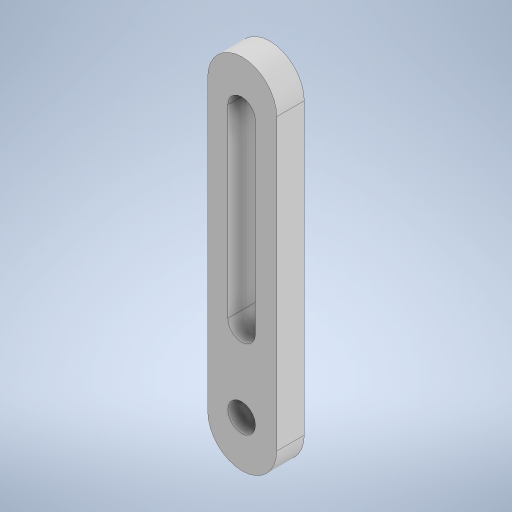
# Autodesk Inventor part: фанерная качалка
Saved by Autodesk Inventor 2023 (Build 270158000, 158)
## iProperties
Created: 2024-03-19
Part Number: фанерная качалка
Material: Типовые
Document SubType Name: Modeling
Designer: liza
Density: 1 g/cm^3
Appearance: По умолчанию
Author: liza
Autodesk Inventor part; units mm, degrees
ref_plane "YZ Plane" through (0, 0, 0) normal (1, 0, 0) x (0, 1, 0)
ref_plane "XZ Plane" through (0, 0, 0) normal (0, 1, 0) x (-1, 0, 0)
ref_plane "XY Plane" through (0, 0, 0) normal (0, 0, 1) x (1, 0, 0)
sketch "Эскиз1" plane through (0, 0, 0) normal (0, 0, 1) x (1, 0, 0)
  arc A0 (7.9627, -8) -> (-2.0373, -8) centre (2.9627, -8) ccw
  line L0 (-2.0373, -8) -> (-2.0373, -50)
  line L1 (7.9627, -8) -> (7.9627, -50)
  arc A1 (-2.0373, -50) -> (7.9627, -50) centre (2.9627, -50) ccw
  dimension "d7" = 42
  dimension "d8" = 5
  constraints: 4 end point, 4 point on circle, 4 tangent, 2 centre point, 2 vertical
  measures "d7" distance of L1.start L1.end
  measures "d8" radius of A1
extrude "Выдавливание1" add sketch "Эскиз1" along normal blind 4
sketch "Эскиз2" plane through (0, 0, 4) normal (0, 0, 1) x (1, 0, 0)
  circle A0 centre (2.8862, -48.3122) radius 2
  arc A1 (4.8862, -10.0339) -> (0.8862, -10.0339) centre (2.8862, -10.0339) ccw
  arc A2 (0.8862, -36.843) -> (4.8862, -36.843) centre (2.8862, -36.843) ccw
  line L0 (0.8862, -10.0339) -> (0.8862, -36.843)
  line L1 (4.8862, -36.843) -> (4.8862, -10.0339)
  point P0 (0, 0)
  dimension "d9" = 4
  dimension "d10" = 4
  dimension "d11" = 4
  constraints: 6 point on circle, 4 end point, 3 centre point, 3 tangent, 2 point on line, 1 parallel
  measures "d9" diameter of A0
  measures "d10" diameter of A1
  measures "d11" diameter of A2
extrude "Выдавливание2" cut sketch "Эскиз2" against normal through all
